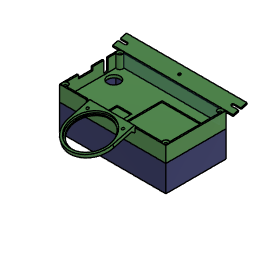
arcade console v12 (Autodesk Fusion 360 archive; units mm, degrees)
design "scatolo"
Autodesk Fusion 360 part; units mm, degrees
(part 1 of 3)
sketch "Schizzo1" plane through (0, 0, 0) normal (0, 0, 1) x (1, 0, 0)
  line L0 (-75, 42.5) -> (75, 42.5)
  line L1 (75, 42.5) -> (75, -42.5)
  line L2 (75, -42.5) -> (-75, -42.5)
  line L3 (-75, -42.5) -> (-75, 42.5)
  line L4 (0, 42.5) -> (0, -42.5) construction
  dimension "d1" = 150
  dimension "d2" = 85
  constraint horizontal L0
  constraint vertical L1
  constraint horizontal L2
  constraint vertical L3
  constraint midpoint L0 L4.start
  constraint midpoint L2 L4.end
  constraint midpoint origin L4
  measures "d1" distance of L0.start L0.end
  measures "d2" distance of L0.start L2.end
extrude "Estrusione1" add sketch "Schizzo1" along normal blind 2 makes body 1
sketch "Schizzo2" plane through (0, 0, 2) normal (0, 0, 1) x (-1, 0, 0)
  line L0 (75, 42.5) -> (-75, 42.5)
  line L1 (-75, 42.5) -> (-75, -42.5)
  line L2 (-75, -42.5) -> (75, -42.5)
  line L3 (75, -42.5) -> (75, 42.5)
  line L4 (75, -42.5) -> (-75, -42.5)
  line L5 (-75, -42.5) -> (-75, 42.5)
  line L6 (-75, 42.5) -> (75, 42.5)
  line L7 (75, 42.5) -> (75, -42.5)
  circle A0 centre (71, -38.5) radius 1
  circle A1 centre (71, -38.5) radius 4
  circle A2 centre (-71, -38.5) radius 1
  circle A3 centre (-71, -38.5) radius 4
  circle A4 centre (71, 38.5) radius 1
  circle A5 centre (71, 38.5) radius 4
  circle A6 centre (-71, 38.5) radius 1
  circle A7 centre (-71, 38.5) radius 4
  line L8 (-73, -40.5) -> (-73, 40.5)
  line L9 (-73, 40.5) -> (73, 40.5)
  line L10 (73, 40.5) -> (73, -40.5)
  line L11 (73, -40.5) -> (-73, -40.5)
  point P0 (-67, -42.5)
  point P1 (-67, -42.5)
  point P2 (75, 34.5)
  point P3 (75, 34.5)
  point P4 (-67, 34.5)
  point P5 (-67, 34.5)
  dimension "d5" = 2
  dimension "d6" = 4
  dimension "d7" = 4
  dimension "d8" = 8
  dimension "d11" = -142
  dimension "d12" = 77
  dimension "d13" = 2
  constraint horizontal L4
  constraint vertical L5
  constraint horizontal L6
  constraint vertical L7
  constraint coincident L0.end L1.start
  constraint coincident L2.end L3.start
  constraint concentric A0 A1
  measures "d5" diameter of A0
  measures "d6" distance of L7 A0.centre
  measures "d7" distance of L4 A0.centre
  measures "d8" diameter of A1
extrude "Estrusione2" add sketch "Schizzo2" along normal blind 35 contours L0 L3 L6 L7 A5 | L0 L6 A5 A7 L9 | A5 L9 L10 | L3 L7 A1 A5 L10 | L0 L1 L5 L6 A7 | A7 L8 L9 | A5 L9 L10 | A1 L10 L11 | L2 L3 L4 L7 A1 | A7 L8 L9 | L1 L5 A3 A7 L8 | A1 L10 L11 | L2 L4 A1 A3 L11 | L1 L2 L4 L5 A3 | A3 L8 L11 | A3 L8 L11 bodies 1
sketch "Schizzo3" plane through (0, 0, 2) normal (0, 0, 1) x (-1, 0, 0)
  arc A0 (-73, 35.0359) -> (-67.5359, 40.5) centre (-71, 38.5) ccw
  line L0 (63.75, -38.5) -> (-63.75, -38.5)
  line L1 (-63.75, -38.5) -> (-63.75, 38.5)
  line L2 (-63.75, 38.5) -> (63.75, 38.5)
  line L3 (63.75, 38.5) -> (63.75, -38.5)
  arc A1 (-67.5359, -40.5) -> (-73, -35.0359) centre (-71, -38.5) ccw
  line L4 (-73, 35.0359) -> (-73, -35.0359)
  arc A2 (67.5359, 40.5) -> (73, 35.0359) centre (71, 38.5) ccw
  line L5 (67.5359, 40.5) -> (-67.5359, 40.5)
  line L6 (-67.5359, -40.5) -> (67.5359, -40.5)
  arc A3 (73, -35.0359) -> (67.5359, -40.5) centre (71, -38.5) ccw
  line L7 (73, -35.0359) -> (73, 35.0359)
  line L8 (0, -38.5) -> (0, 38.5) construction
  dimension "d16" = 127.5
  dimension "d17" = 77
  constraint horizontal L0
  constraint vertical L1
  constraint horizontal L2
  constraint vertical L3
  constraint midpoint L0 L8.start
  constraint midpoint L2 L8.end
  constraint midpoint origin L8
  measures "d16" distance of L0.start L0.end
  measures "d17" distance of L0.start L2.end
extrude "Estrusione3" add sketch "Schizzo3" along normal blind 2 bodies 1
sketch "Schizzo4" plane through (0, 40.5, 0) normal (0, -1, 0) x (1, 0, 0)
  line L0 (-67.5359, 4) -> (67.5359, 4)
  line L1 (67.5359, 4) -> (67.5359, 37)
  line L2 (67.5359, 37) -> (-67.5359, 37)
  line L3 (-67.5359, 37) -> (-67.5359, 4)
  circle A0 centre (48.6233, 33.35) radius 3.65
  line L4 (44.9733, 33.35) -> (52.2733, 33.35)
  line L5 (52.2733, 33.35) -> (52.2733, 37)
  line L6 (52.2733, 37) -> (44.9733, 37)
  line L7 (44.9733, 37) -> (44.9733, 33.35)
  dimension "d20" = 7.3
  constraint horizontal L4
  constraint vertical L5
  constraint horizontal L6
  constraint vertical L7
  constraint tangent A0 L7
  constraint tangent A0 L6
  constraint tangent A0 L5
  constraint midpoint A0.centre L4
  constraint collinear L2 L6
  measures "d20" diameter of A0
extrude "Estrusione4" cut sketch "Schizzo4" against normal blind 16.479 contours L2 A0 L6 L7 | L2 A0 L5 L6 | A0 L4 | A0 L4 bodies 1
sketch "Schizzo5" plane through (0, 0, 37) normal (0, 0, 1) x (-1, 0, 0)
  line L0 (-52.2733, -42.5) -> (-52.2733, -40.5)
  line L1 (-52.2733, -40.5) -> (-67.5359, -40.5)
  arc A0 (-67.5359, -40.5) -> (-73, -35.0359) centre (-71, -38.5) ccw
  line L2 (-73, -35.0359) -> (-73, 35.0359)
  arc A1 (-73, 35.0359) -> (-67.5359, 40.5) centre (-71, 38.5) ccw
  line L3 (-67.5359, 40.5) -> (67.5359, 40.5)
  arc A2 (67.5359, 40.5) -> (73, 35.0359) centre (71, 38.5) ccw
  line L4 (73, 35.0359) -> (73, -35.0359)
  arc A3 (73, -35.0359) -> (67.5359, -40.5) centre (71, -38.5) ccw
  line L5 (67.5359, -40.5) -> (-44.9733, -40.5)
  line L6 (-44.9733, -40.5) -> (-44.9733, -42.5)
  line L7 (-44.9733, -42.5) -> (75, -42.5)
  line L8 (75, -42.5) -> (75, 42.5)
  line L9 (75, 42.5) -> (-75, 42.5)
  line L10 (-75, 42.5) -> (-75, -42.5)
  line L11 (-75, -42.5) -> (-52.2733, -42.5)
  circle A4 centre (-71, 38.5) radius 1
  circle A5 centre (71, -38.5) radius 1
  circle A6 centre (71, 38.5) radius 1
  circle A7 centre (-71, -38.5) radius 1
  circle A8 centre (-71, 38.5) radius 2
  circle A9 centre (71, 38.5) radius 2
  circle A10 centre (71, -38.5) radius 2
  circle A11 centre (-71, -38.5) radius 2
  line L12 (-44.9733, -42.5) -> (-52.2733, -42.5)
  dimension "d23" = 4
  dimension "d24" = 4
  dimension "d25" = 4
  dimension "d26" = 4
  constraint concentric A1 A8
  constraint concentric A2 A9
  constraint concentric A3 A10
  constraint concentric A0 A11
  constraint coincident L6.end L7.start
  constraint coincident L0.start L11.end
  measures "d23" diameter of A8
  measures "d24" diameter of A9
  measures "d25" diameter of A10
  measures "d26" diameter of A11
extrude "Estrusione1'" add sketch "Schizzo5" along normal blind 2 separate body contours L0 L1 A0 L2 A1 L3 A2 L4 A3 L5 L6 L7 L8 L9 L10 L11 | L0 L1 A0 L2 A1 L3 A2 L4 A3 L5 L6 L12 makes body 2 in component "sopra"
sketch "Schizzo6" plane through (0, 0, 39) normal (0, 0, 1) x (-1, 0, 0)
  circle A0 centre (-71, 38.5) radius 2
  circle A1 centre (-71, -38.5) radius 2
  circle A2 centre (71, -38.5) radius 2
  circle A3 centre (71, 38.5) radius 2
  line L0 (75, -42.5) -> (75, 42.5)
  line L1 (75, 42.5) -> (-75, 42.5)
  line L2 (-75, 42.5) -> (-75, -42.5)
  line L3 (-75, -42.5) -> (75, -42.5)
  line L4 (-52.2733, -42.5) -> (-52.2733, -40.5)
  line L5 (-52.2733, -40.5) -> (-67.5359, -40.5)
  arc A4 (-67.5359, -40.5) -> (-73, -35.0359) centre (-71, -38.5) ccw
  line L6 (-73, -35.0359) -> (-73, 35.0359)
  arc A5 (-73, 35.0359) -> (-67.5359, 40.5) centre (-71, 38.5) ccw
  line L7 (-67.5359, 40.5) -> (67.5359, 40.5)
  arc A6 (67.5359, 40.5) -> (73, 35.0359) centre (71, 38.5) ccw
  line L8 (73, 35.0359) -> (73, -35.0359)
  arc A7 (73, -35.0359) -> (67.5359, -40.5) centre (71, -38.5) ccw
  line L9 (67.5359, -40.5) -> (-44.9733, -40.5)
  line L10 (-44.9733, -40.5) -> (-44.9733, -42.5)
  line L11 (-44.9733, -42.5) -> (75, -42.5)
  line L12 (75, -42.5) -> (75, 42.5)
  line L13 (75, 42.5) -> (-75, 42.5)
  line L14 (-75, 42.5) -> (-75, -42.5)
  line L15 (-75, -42.5) -> (-52.2733, -42.5)
  circle A8 centre (-71, 38.5) radius 1
  circle A9 centre (71, -38.5) radius 1
  circle A10 centre (71, 38.5) radius 1
  circle A11 centre (-71, -38.5) radius 1
  line L16 (-52.2733, -40.5) -> (-44.9733, -40.5)
  line L17 (-44.9733, -40.5) -> (-44.9733, -42.5)
  line L18 (-44.9733, -42.5) -> (-52.2733, -42.5)
  line L19 (-52.2733, -42.5) -> (-52.2733, -40.5)
  constraint horizontal L16
  constraint vertical L17
  constraint horizontal L18
  constraint vertical L19
  constraint coincident L10.end L11.start
  constraint coincident L4.end L5.start
extrude "Estrusione2'" add sketch "Schizzo6" along normal blind 20 contours L0 L1 L2 L3 L4 L5 A4 L6 A5 L7 A6 L8 A7 L9 L10 L11 L12 L13 L14 L15 L17 L19 | L3 L4 L10 L16 L17 L18 L19 bodies 2 in component "sopra"
sketch "Schizzo7" plane through (0, 0, 39) normal (0, 0, 1) x (-1, 0, 0)
  arc A0 (73, -35.0359) -> (67.5359, -40.5) centre (71, -38.5) ccw
  line L0 (73, -35.0359) -> (73, 35.0359)
  arc A1 (67.5359, 40.5) -> (73, 35.0359) centre (71, 38.5) ccw
  line L1 (67.5359, 40.5) -> (-67.5359, 40.5)
  arc A2 (-73, 35.0359) -> (-67.5359, 40.5) centre (-71, 38.5) ccw
  line L2 (-73, 35.0359) -> (-73, -35.0359)
  arc A3 (-67.5359, -40.5) -> (-73, -35.0359) centre (-71, -38.5) ccw
  line L3 (-67.5359, -40.5) -> (67.5359, -40.5)
  circle A4 centre (60, -19) radius 9
  dimension "d31" = 18
  measures "d31" diameter of A4
extrude "Estrusione3'" cut sketch "Schizzo7" against normal blind 8.932 contours A4 bodies 2 in component "sopra"
sketch "Schizzo8" plane through (0, 40.5, 0) normal (0, -1, 0) x (1, 0, 0)
  line L0 (-67.5359, 39) -> (67.5359, 39)
  line L1 (67.5359, 39) -> (67.5359, 59)
  line L2 (67.5359, 59) -> (-67.5359, 59)
  line L3 (-67.5359, 59) -> (-67.5359, 39)
sketch "Schizzo9" plane through (0, 0, 39) normal (0, 0, 1) x (-1, 0, 0)
  circle A0 centre (60, -19) radius 9
  arc A1 (73, -35.0359) -> (67.5359, -40.5) centre (71, -38.5) ccw
  line L0 (73, -35.0359) -> (73, 35.0359)
  arc A2 (67.5359, 40.5) -> (73, 35.0359) centre (71, 38.5) ccw
  line L1 (67.5359, 40.5) -> (-67.5359, 40.5)
  arc A3 (-73, 35.0359) -> (-67.5359, 40.5) centre (-71, 38.5) ccw
  line L2 (-73, 35.0359) -> (-73, -35.0359)
  arc A4 (-67.5359, -40.5) -> (-73, -35.0359) centre (-71, -38.5) ccw
  line L3 (-67.5359, -40.5) -> (67.5359, -40.5)
  circle A5 centre (-23.6081, -24.9772) radius 0.254
  line L4 (-46.4381, -12.0232) -> (-46.4381, 20.7428)
  line L5 (22.1119, 25.8228) -> (22.1119, -27.5557)
  circle A6 centre (0.7459, -24.9772) radius 0.254
  circle A7 centre (-15.9881, 23.2828) radius 0.254
  circle A8 centre (-26.1481, -24.9772) radius 0.254
  circle A9 centre (-33.7681, 23.2828) radius 0.254
  circle A10 centre (-41.3881, -24.9772) radius 0.254
  circle A11 centre (-13.4481, 23.2828) radius 0.254
  circle A12 centre (-28.6881, 23.2828) radius 0.254
  circle A13 centre (-5.8281, 23.2828) radius 0.254
  circle A14 centre (-31.2281, 23.2828) radius 0.254
  line L6 (-43.9581, 25.8228) -> (22.1119, 25.8228)
  line L7 (-43.9581, 25.8228) -> (-43.9581, 23.2828)
  circle A15 centre (-1.7941, -24.9772) radius 0.254
  line L8 (-43.9581, -14.5632) -> (-46.4381, -12.0232)
  circle A16 centre (-38.8481, 23.2828) radius 0.254
  circle A17 centre (-11.9541, -24.9772) radius 0.254
  circle A18 centre (-10.9081, 23.2828) radius 0.254
  circle A19 centre (-9.4141, -24.9772) radius 0.254
  circle A20 centre (3.2859, -24.9772) radius 0.254
  circle A21 centre (-18.5281, 23.2828) radius 0.254
  circle A22 centre (-19.5741, -24.9772) radius 0.254
  line L9 (-46.4381, 20.7428) -> (-43.9581, 23.2828)
  circle A23 centre (-23.6081, 23.2828) radius 0.254
  circle A24 centre (-14.4941, -24.9772) radius 0.254
  circle A25 centre (-4.3341, -24.9772) radius 0.254
  line L10 (-43.9581, -25.9909) -> (-42.3933, -27.5557)
  line L11 (-42.3933, -27.5557) -> (22.1119, -27.5557)
  circle A26 centre (-31.2281, -24.9772) radius 0.254
  circle A27 centre (-6.8741, -24.9772) radius 0.254
  circle A28 centre (-36.3081, -24.9772) radius 0.254
  circle A29 centre (-17.0341, -24.9772) radius 0.254
  circle A30 centre (-41.3881, 23.2828) radius 0.254
  circle A31 centre (-38.8481, -24.9772) radius 0.254
  circle A32 centre (-28.6881, -24.9772) radius 0.254
  circle A33 centre (-33.7681, -24.9772) radius 0.254
  circle A34 centre (-36.3081, 23.2828) radius 0.254
  circle A35 centre (8.1419, 23.2828) radius 1.5875
  circle A36 centre (-43.9581, -9.7372) radius 1.5875
  circle A37 centre (-21.0681, 23.2828) radius 0.254
  circle A38 centre (6.8419, -24.9772) radius 1.5875
  circle A39 centre (-43.9581, 18.2028) radius 1.5875
  circle A40 centre (-8.3681, 23.2828) radius 0.254
  line L12 (-43.9581, -25.9909) -> (-43.9581, -14.5632)
  circle A41 centre (-45.7728, -24.3932) radius 0.254
  line L13 (-68.6028, -11.4392) -> (-68.6028, 21.3268)
  line L14 (-0.0528, 26.4068) -> (-0.0528, -26.9717)
  circle A42 centre (-21.4188, -24.3932) radius 0.254
  circle A43 centre (-38.1528, 23.8668) radius 0.254
  circle A44 centre (-48.3128, -24.3932) radius 0.254
  circle A45 centre (-55.9328, 23.8668) radius 0.254
  circle A46 centre (-63.5528, -24.3932) radius 0.254
  circle A47 centre (-35.6128, 23.8668) radius 0.254
  circle A48 centre (-50.8528, 23.8668) radius 0.254
  circle A49 centre (-27.9928, 23.8668) radius 0.254
  circle A50 centre (-53.3928, 23.8668) radius 0.254
  line L15 (-66.1228, 26.4068) -> (-0.0528, 26.4068)
  line L16 (-66.1228, 26.4068) -> (-66.1228, 23.8668)
  circle A51 centre (-23.9588, -24.3932) radius 0.254
  line L17 (-66.1228, -13.9792) -> (-68.6028, -11.4392)
  circle A52 centre (-61.0128, 23.8668) radius 0.254
  circle A53 centre (-34.1188, -24.3932) radius 0.254
  circle A54 centre (-33.0728, 23.8668) radius 0.254
  circle A55 centre (-31.5788, -24.3932) radius 0.254
  circle A56 centre (-18.8788, -24.3932) radius 0.254
  circle A57 centre (-40.6928, 23.8668) radius 0.254
  circle A58 centre (-41.7388, -24.3932) radius 0.254
  line L18 (-68.6028, 21.3268) -> (-66.1228, 23.8668)
  circle A59 centre (-45.7728, 23.8668) radius 0.254
  circle A60 centre (-36.6588, -24.3932) radius 0.254
  circle A61 centre (-26.4988, -24.3932) radius 0.254
  line L19 (-66.1228, -25.4069) -> (-64.558, -26.9717)
  line L20 (-64.558, -26.9717) -> (-0.0528, -26.9717)
  circle A62 centre (-53.3928, -24.3932) radius 0.254
  circle A63 centre (-29.0388, -24.3932) radius 0.254
  circle A64 centre (-58.4728, -24.3932) radius 0.254
  circle A65 centre (-39.1988, -24.3932) radius 0.254
  circle A66 centre (-63.5528, 23.8668) radius 0.254
  circle A67 centre (-61.0128, -24.3932) radius 0.254
  circle A68 centre (-50.8528, -24.3932) radius 0.254
  circle A69 centre (-55.9328, -24.3932) radius 0.254
  circle A70 centre (-58.4728, 23.8668) radius 0.254
  circle A71 centre (-14.0228, 23.8668) radius 1.5875
  circle A72 centre (-66.1228, -9.1532) radius 1.5875
  circle A73 centre (-43.2328, 23.8668) radius 0.254
  circle A74 centre (-15.3228, -24.3932) radius 1.5875
  circle A75 centre (-66.1228, 18.7868) radius 1.5875
  circle A76 centre (-30.5328, 23.8668) radius 0.254
  line L21 (-66.1228, -25.4069) -> (-66.1228, -13.9792)
  dimension "d34" = 50.8881
  measures "d34" distance of L0 L5
extrude "Estrusione4'" add sketch "Schizzo9" along normal blind 2 contours A1 L0 A2 L1 A3 L2 A4 L3 | L5 L6 L10 L11 L14 L20 | A6 | A20 | A35 | A38 bodies 2 in component "sopra"
sketch "Schizzo10" plane through (0, 0, 39) normal (0, 0, 1) x (-1, 0, 0)
  line L0 (-0.0528, -26.9717) -> (-0.0528, 26.4068)
  line L1 (-0.0528, 26.4068) -> (-66.1228, 26.4068)
  line L2 (-66.1228, 26.4068) -> (-66.1228, 23.8668)
  line L3 (-66.1228, 23.8668) -> (-68.6028, 21.3268)
  line L4 (-68.6028, 21.3268) -> (-68.6028, -11.4392)
  line L5 (-68.6028, -11.4392) -> (-66.1228, -13.9792)
  line L6 (-66.1228, -13.9792) -> (-66.1228, -25.4069)
  line L7 (-66.1228, -25.4069) -> (-64.558, -26.9717)
  line L8 (-64.558, -26.9717) -> (-0.0528, -26.9717)
  line L9 (0.4472, 26.9068) -> (-66.6228, 26.9068)
  line L10 (-66.6228, 26.9068) -> (-66.6228, 24.0704)
  line L11 (-66.6228, 24.0704) -> (-69.1028, 21.5304)
  line L12 (-69.1028, 21.5304) -> (-69.1028, -11.6428)
  line L13 (-69.1028, -11.6428) -> (-66.6228, -14.1828)
  line L14 (-66.6228, -14.1828) -> (-66.6228, -25.614)
  line L15 (-66.6228, -25.614) -> (-64.7651, -27.4717)
  line L16 (-64.7651, -27.4717) -> (0.4472, -27.4717)
  line L17 (0.4472, -27.4717) -> (0.4472, 26.9068)
  dimension "d37" = 0.5
extrude "Estrusione5" cut sketch "Schizzo10" along normal blind 34.396 bodies 2 in component "sopra"
ref_plane "Piano di lavoro1" through (0, 0, 48) normal (-1, 0, 0) x (0, -1, 0)
sketch "Schizzo12" plane through (0, 0, 0) normal (-1, 0, 0) x (0, -1, 0)
  line L0 (-42.5, 37) -> (42.5, 37) construction
  line L1 (42.5, 37) -> (42.5, 59) construction
  line L2 (42.5, 59) -> (-42.5, 59) construction
  line L3 (-42.5, 59) -> (-42.5, 37) construction
  line L4 (-42.5, 59) -> (-61.8185, 64.1764)
  line L5 (-42.5, 59) -> (-22.5, 59) construction
  line L6 (-61.8185, 64.1764) -> (-62.3362, 62.2445)
  line L7 (-62.3362, 62.2445) -> (-42.5, 56.9294)
  line L8 (-42.5, 59) -> (-42.5, 56.9294)
  dimension "d40" = 165
  dimension "d41" = 20
  dimension "d42" = 2
  constraint horizontal L5
  constraint coincident L2.end L3.start
  constraint perpendicular L4 L6
  constraint perpendicular L6 L7
  constraint perpendicular L2 L8
  constraint coincident L3 L7.end
  measures "d40" angle of L4 L5
  measures "d41" distance of L2.end L4.end
  measures "d42" distance of L4.end L6.end
extrude "Estrusione6" add sketch "Schizzo12" along normal mid plane 170 bodies 2 in component "sopra"
sketch "Schizzo13" plane through (0, -11.903, 44.4227) normal (0, -0.258819, 0.965926) x (1, 0, 0)
  line L0 (85, 76.3222) -> (-85, 76.3222)
  line L1 (-85, 76.3222) -> (-85, 56.3222)
  line L2 (-85, 56.3222) -> (-75, 56.3222)
  line L3 (-75, 56.3222) -> (75, 56.3222)
  line L4 (75, 56.3222) -> (85, 56.3222)
  line L5 (85, 56.3222) -> (85, 76.3222)
  line L6 (-85, 76.3222) -> (85, 76.3222) construction
  line L7 (-85, 65.8222) -> (85, 65.8222) construction
  circle A0 centre (-75, 65.8222) radius 1.75
  line L8 (-85, 67.5722) -> (-75, 67.5722)
  line L9 (-75, 67.5722) -> (-75, 64.0722)
  line L10 (-75, 64.0722) -> (-85, 64.0722)
  line L11 (-85, 64.0722) -> (-85, 67.5722)
  circle A1 centre (0, 65.8222) radius 1.75
  circle A2 centre (75, 65.8222) radius 1.75
  line L12 (85, 67.5722) -> (75, 67.5722)
  line L13 (75, 67.5722) -> (75, 64.0722)
  line L14 (75, 64.0722) -> (85, 64.0722)
  line L15 (85, 64.0722) -> (85, 67.5722)
  dimension "d45" = 9.5
  dimension "d46" = 3.5
  dimension "d47" = 3.5
  dimension "d48" = 3.5
  dimension "d49" = 10
  dimension "d50" = 10
  constraint coincident L1 L7.start
  constraint coincident L5 L7.end
  constraint perpendicular L5 L7
  constraint coincident L7 A0.centre
  constraint horizontal L8
  constraint vertical L9
  constraint horizontal L10
  constraint vertical L11
  constraint midpoint L7 A1.centre
  constraint coincident L7 A2.centre
  constraint horizontal L12
  constraint vertical L13
  constraint horizontal L14
  constraint vertical L15
  constraint collinear L5 L15
  constraint collinear L1 L11
  constraint midpoint A2.centre L13
  constraint midpoint A0.centre L9
  constraint tangent A0 L8
  constraint tangent A2 L12
  measures "d45" distance of L2 L7
  measures "d46" diameter of A0
  measures "d47" diameter of A1
  measures "d48" diameter of A2
  measures "d49" distance of L8.start L8.end
  measures "d50" distance of L12.start L12.end
extrude "Estrusione7" cut sketch "Schizzo13" against normal blind 2.904 contours L5 A2 L12 L14 L15 | L1 A0 L8 L10 L11 | A2 L13 | A2 L13 | A0 L9 | A0 L9 | A1 bodies 2 in component "sopra"
sketch "Schizzo14" plane through (0, 0, 0) normal (-1, 0, 0) x (0, -1, 0)
  line L0 (43.4059, 62.3807) -> (42.5, 59)
  line L1 (43.4059, 62.3807) -> (46.9059, 62.3807) construction
  line L2 (42.5, 37) -> (-42.5, 37) construction
  line L3 (-42.5, 37) -> (-42.5, 56.9294) construction
  line L4 (-42.5, 56.9294) -> (-42.5, 59) construction
  line L5 (-42.5, 59) -> (42.5, 59) construction
  line L6 (42.5, 59) -> (42.5, 37) construction
  line L7 (43.4059, 62.3807) -> (104.2592, 46.0751)
  line L8 (43.4059, 62.3807) -> (106.4059, 62.3807) construction
  line L9 (104.2592, 46.0751) -> (102.9651, 41.2455)
  line L10 (102.9651, 41.2455) -> (42.5, 57.4471)
  line L11 (42.5, 59) -> (42.5, 57.4471)
  line L12 (-34.5, 59) -> (-40.5, 59) construction
  line L13 (-35.0359, 59) -> (35.0359, 59) construction
  line L14 (40.5, 59) -> (34.5, 59) construction
  line L15 (40.5, 59) -> (34.5, 59) construction
  line L16 (35.0359, 59) -> (-35.0359, 59) construction
  line L17 (-34.5, 59) -> (-40.5, 59) construction
  line L18 (36.5, 59) -> (40.5, 59) construction
  line L19 (-40.5, 59) -> (-36.5, 59) construction
  line L20 (-40.5, 59) -> (-36.5, 59) construction
  line L21 (36.5, 59) -> (40.5, 59) construction
  line L22 (-42.5, 59) -> (42.5, 59) construction
  line L23 (42.5, 59) -> (-42.5, 59) construction
  line L24 (40.5, 59) -> (43.4059, 62.3807)
  line L25 (42.5, 59) -> (40.5, 59)
  dimension "d53" = 105
  dimension "d54" = 3.5
  dimension "d55" = 15
  dimension "d56" = 63
  dimension "d57" = 5
  constraint horizontal L1
  constraint coincident L0.end L5.end
  constraint horizontal L8
  constraint perpendicular L7 L9
  constraint perpendicular L9 L10
  constraint perpendicular L5 L11
  constraint coincident L6 L10.end
  constraint coincident L14.start L15.start
  measures "d53" angle of L0 L1
  measures "d54" distance of L0.start L0.end
  measures "d55" angle of L7 L8
  measures "d56" distance of L0.start L7.end
  measures "d57" distance of L7.end L9.end
extrude "Estrusione8" add sketch "Schizzo14" along normal mid plane 63 bodies 2 in component "sopra"
chamfer "Smusso1" distance 5 angle 45 1 edges at (0, -42.5, 57.4471) on bodies 2 in component "sopra"
sketch "Schizzo15" plane through (0, -18.5028, 69.0535) normal (0, -0.258819, 0.965926) x (1, 0, 0)
  line L0 (31.5, -25.7815) -> (-31.5, -25.7815)
  line L1 (-31.5, -25.7815) -> (-31.5, -88.7815)
  line L2 (-31.5, -88.7815) -> (31.5, -88.7815)
  line L3 (31.5, -88.7815) -> (31.5, -25.7815)
  circle A0 centre (0, -57.2815) radius 28.5
  line L4 (-31.5, -85.7815) -> (31.5, -85.7815) construction
  line L5 (31.5, -85.7815) -> (31.5, -88.7815) construction
  line L6 (31.5, -88.7815) -> (-31.5, -88.7815) construction
  line L7 (-31.5, -88.7815) -> (-31.5, -85.7815) construction
  line L8 (-63.75, -36.6705, -59.593) -> (63.75, -36.6705, -59.593) construction
  line L9 (0, -85.7815) -> (0, -112) construction
  dimension "d61" = 57
  dimension "d62" = 3
  constraint horizontal L4
  constraint vertical L5
  constraint horizontal L6
  constraint vertical L7
  constraint collinear L2 L6
  constraint tangent A0 L4
  constraint collinear L3 L5
  constraint collinear L1 L7
  constraint midpoint L4 L9.start
  constraint perpendicular L4 L9
  constraint coincident A0.centre L9
  measures "d61" diameter of A0
  measures "d62" distance of L4.start L1.end
extrude "Estrusione9" cut sketch "Schizzo15" against normal blind 3 contours A0 bodies 2 in component "sopra"
sketch "Schizzo16" plane through (0, -17.7264, 66.1557) normal (0, -0.258819, 0.965926) x (1, 0, 0)
  circle A0 centre (0, -57.2815) radius 28.5
  circle A1 centre (0, -57.2815) radius 26.5
  dimension "d65" = 53
  constraint concentric A0 A1
  measures "d65" diameter of A1
extrude "Estrusione10" cut sketch "Schizzo16" against normal blind 2.232 contours A1 bodies 2 in component "sopra"
sketch "Schizzo17" plane through (0, 0, 41) normal (0, 0, 1) x (-1, 0, 0)
  line L0 (0.4472, -27.4717) -> (-64.7651, -27.4717)
  line L1 (-64.7651, -27.4717) -> (-66.6228, -25.614)
  line L2 (-66.6228, -25.614) -> (-66.6228, -14.1828)
  line L3 (-66.6228, -14.1828) -> (-69.1028, -11.6428)
  line L4 (-69.1028, -11.6428) -> (-69.1028, 21.5304)
  line L5 (-69.1028, 21.5304) -> (-66.6228, 24.0704)
  line L6 (-66.6228, 24.0704) -> (-66.6228, 26.9068)
  line L7 (-66.6228, 26.9068) -> (0.4472, 26.9068)
  line L8 (0.4472, 26.9068) -> (0.4472, -27.4717)
  circle A0 centre (60, -19) radius 9
  line L9 (-73, 35.0359) -> (-73, -35.0359)
  arc A1 (-67.5359, -40.5) -> (-73, -35.0359) centre (-71, -38.5) ccw
  line L10 (-67.5359, -40.5) -> (67.5359, -40.5)
  arc A2 (73, -35.0359) -> (67.5359, -40.5) centre (71, -38.5) ccw
  line L11 (73, -35.0359) -> (73, 35.0359)
  arc A3 (67.5359, 40.5) -> (73, 35.0359) centre (71, 38.5) ccw
  line L12 (67.5359, 40.5) -> (-67.5359, 40.5)
  arc A4 (-73, 35.0359) -> (-67.5359, 40.5) centre (-71, 38.5) ccw
  line L13 (26.4472, 9.9068) -> (5.4472, 9.9068)
  line L14 (5.4472, 9.9068) -> (5.4472, 26.9068)
  line L15 (5.4472, 26.9068) -> (26.4472, 26.9068)
  line L16 (26.4472, 26.9068) -> (26.4472, 9.9068)
  dimension "d68" = 5
  dimension "d69" = 21
  dimension "d70" = 17
  constraint horizontal L13
  constraint vertical L14
  constraint horizontal L15
  constraint vertical L16
  constraint collinear L7 L15
  measures "d68" distance of L8 L14
  measures "d69" distance of L13.start L13.end
  measures "d70" distance of L13.start L15.end
extrude "Estrusione11" cut sketch "Schizzo17" against normal blind 2 contours L13 L14 L15 L16 bodies 2 in component "sopra"
sketch "Schizzo18" plane through (0, -42.5, 0) normal (0, -1, 0) x (1, 0, 0)
  line L0 (-31.5, 52.4471) -> (-31.5, 59)
  line L1 (-31.5, 59) -> (-75, 59)
  line L2 (-75, 59) -> (-75, 37)
  line L3 (-75, 37) -> (75, 37)
  line L4 (75, 37) -> (75, 59)
  line L5 (75, 59) -> (31.5, 59)
  line L6 (31.5, 59) -> (31.5, 52.4471)
  line L7 (31.5, 52.4471) -> (-31.5, 52.4471)
  circle A0 centre (-35.6271, 49) radius 1.5
  line L8 (-37.1271, 59) -> (-34.1271, 59)
  line L9 (-34.1271, 59) -> (-34.1271, 49)
  line L10 (-34.1271, 49) -> (-37.1271, 49)
  line L11 (-37.1271, 49) -> (-37.1271, 59)
  dimension "d73" = 3
  dimension "d74" = 3
  dimension "d75" = 10
  constraint horizontal L8
  constraint vertical L9
  constraint horizontal L10
  constraint vertical L11
  constraint collinear L1 L8
  constraint midpoint A0.centre L10
  measures "d73" diameter of A0
  measures "d74" distance of L8.start L8.end
  measures "d75" distance of L8.start L10.end
extrude "Estrusione12" cut sketch "Schizzo18" against normal blind 5.663 contours L1 A0 L8 L9 L11 | A0 L10 | A0 L10 bodies 2 in component "sopra"
fillet "Raccordo1" radius 31.5 2 edges at (-31.5, -103.6121, 43.6603) (31.5, -103.6121, 43.6603) on bodies 2 in component "sopra"
sketch "Schizzo19" plane through (0, -18.5028, 69.0535) normal (0, -0.258819, 0.965926) x (1, 0, 0)
  arc A0 (-31.5, -57.2815) -> (31.5, -57.2815) centre (0, -57.2815) ccw
  line L0 (31.5, -57.2815) -> (31.5, -25.7815)
  line L1 (31.5, -25.7815) -> (-31.5, -25.7815)
  line L2 (-31.5, -25.7815) -> (-31.5, -57.2815)
  circle A1 centre (0, -57.2815) radius 28.5
  circle A2 centre (-25, -35.7815) radius 1.75
  circle A3 centre (25, -35.7815) radius 1.75
  line L3 (-25, -35.7815) -> (25, -35.7815)
  line L4 (0, -25.7815) -> (0, -35.7815)
  dimension "d80" = 3.5
  dimension "d81" = 3.5
  dimension "d82" = 50
  dimension "d85" = 10
  constraint coincident A2.centre L3.start
  constraint parallel L1 L3
  constraint midpoint L1 L4.start
  constraint midpoint L3 L4.end
  constraint vertical L4
  constraint coincident A3.centre L3.end
  measures "d80" diameter of A2
  measures "d81" diameter of A3
  measures "d82" distance of A2.centre A3.centre
  measures "d85" distance of L4.start L4.end
extrude "Estrusione13" cut sketch "Schizzo19" against normal blind 6.961 contours A2 | A3 bodies 2 in component "sopra"
copy_body "Corpo->Comp1" bodies 1 removing the originals makes body 3 in component "sotto"
chamfer "Smusso2" distance 1.8 angle 45 4 edges at (-69.1353, 37.7768, 59) (-69.1353, -39.2232, 59) (72.8647, 37.7768, 59) (72.8647, -39.2232, 59) on bodies 2 in component "sopra"
sketch "Schizzo20" plane through (-75, 0, 0) normal (-1, 0, 0) x (0, -1, 0)
  line L0 (-42.5, 37) -> (42.5, 37)
  line L1 (42.5, 37) -> (42.5, 59)
  line L2 (42.5, 59) -> (-42.5, 59)
  line L3 (-42.5, 59) -> (-42.5, 56.9294)
  line L4 (-42.5, 56.9294) -> (-42.5, 37)
  circle A0 centre (-20.9777, 44) radius 3
  line L5 (-23.9777, 59) -> (-17.9777, 59)
  line L6 (-17.9777, 59) -> (-17.9777, 44)
  line L7 (-17.9777, 44) -> (-23.9777, 44)
  line L8 (-23.9777, 44) -> (-23.9777, 59)
  line L9 (-26.9777, 59) -> (-14.9777, 59)
  line L10 (-14.9777, 59) -> (-14.9777, 47)
  line L11 (-14.9777, 47) -> (-26.9777, 47)
  line L12 (-26.9777, 47) -> (-26.9777, 59)
  dimension "d87" = 6
  dimension "d88" = 6
  dimension "d89" = 15
  dimension "d95" = 12
  dimension "d96" = 12
  constraint horizontal L5
  constraint vertical L6
  constraint horizontal L7
  constraint vertical L8
  constraint midpoint A0.centre L7
  constraint collinear L2 L5
  constraint horizontal L9
  constraint vertical L10
  constraint horizontal L11
  constraint vertical L12
  constraint midpoint L5 L9
  measures "d87" diameter of A0
  measures "d88" distance of L5.start L5.end
  measures "d89" distance of L5.start L7.end
  measures "d95" distance of L9.start L9.end
  measures "d96" distance of L9.start L11.end
extrude "Estrusione14" cut sketch "Schizzo20" against normal blind 5.067 contours L2 L5 L6 L8 L9 L11 | A0 L6 L11 | A0 L8 L11 | A0 L7 | A0 L7 bodies 2 in component "sopra"
sketch "Schizzo21" plane through (0, 0, 59) normal (0, 0, 1) x (-1, 0, 0)
  line L0 (73, -17.9777) -> (75, -17.9777)
  line L1 (75, -17.9777) -> (75, 42.5)
  line L2 (75, 42.5) -> (37.1271, 42.5)
  line L3 (37.1271, 42.5) -> (37.1271, 40.5)
  line L4 (37.1271, 40.5) -> (67.5359, 40.5)
  arc A0 (67.5359, 40.5) -> (73, 35.0359) centre (71, 38.5) ccw
  line L5 (73, 35.0359) -> (73, -17.9777)
  circle A1 centre (71, 38.5) radius 3.8
  line L6 (83.0164, -2.2982) -> (65.8423, -2.2982)
  line L7 (65.8423, -2.2982) -> (65.8423, 17.7018)
  line L8 (65.8423, 17.7018) -> (83.0164, 17.7018)
  line L9 (83.0164, 17.7018) -> (83.0164, -2.2982)
  dimension "d92" = 20
  constraint horizontal L6
  constraint vertical L7
  constraint horizontal L8
  constraint vertical L9
  measures "d92" distance of L6.start L8.end
extrude "Estrusione15" cut sketch "Schizzo21" against normal blind 5 contours L1 L5 L6 L8 bodies 2 in component "sopra"
component "sopra" placed x (1, 0, 0) y (0, 1, 0) z (0, 0, 1) at (0, 0, 0)
component "sotto" placed x (1, 0, 0) y (0, 1, 0) z (0, 0, 1) at (0, 0, 0)
equation "d40 = 180 deg - 15 deg"
equation "d53 = 90 deg + 15 deg"
equation "d56 = 57 mm + 6 mm"
equation "d58 = 57 mm + 6 mm"
equation "d79 = ( ( 57 + 6 ) / 2 ) * 1 mm"

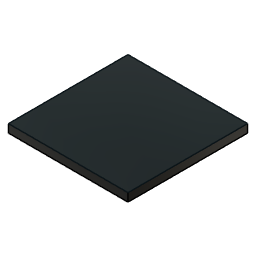
design "display 32x32"
Autodesk Fusion 360 part; units mm, degrees
sketch "Schizzo1" plane through (0, 0, 0) normal (0, 0, 1) x (1, 0, 0)
  line L0 (-96, 96) -> (96, 96)
  line L1 (96, 96) -> (96, -96)
  line L2 (96, -96) -> (-96, -96)
  line L3 (-96, -96) -> (-96, 96)
  line L4 (0, 96) -> (0, -96) construction
  dimension "d1" = 192
  dimension "d2" = 192
  constraint horizontal L0
  constraint vertical L1
  constraint horizontal L2
  constraint vertical L3
  constraint midpoint L0 L4.start
  constraint midpoint L2 L4.end
  constraint midpoint origin L4
  measures "d1" distance of L0.start L0.end
  measures "d2" distance of L0.start L2.end
extrude "Estrusione1" add sketch "Schizzo1" along normal blind 13.2 makes body 1
sketch "Schizzo2" plane through (0, 0, 13.2) normal (0, 0, 1) x (-1, 0, 0)
  line L0 (96, 96) -> (-96, 96)
  line L1 (-96, 96) -> (-96, -96)
  line L2 (-96, -96) -> (96, -96)
  line L3 (96, -96) -> (96, 96)
sketch "Schizzo3" plane through (0, 0, 0) normal (0, 0, -1) x (1, 0, 0)
  line L0 (96, 96) -> (-96, 96)
  line L1 (-96, 96) -> (-96, -96)
  line L2 (-96, -96) -> (96, -96)
  line L3 (96, -96) -> (96, 96)
  circle A0 centre (86.5, 0) radius 0.5
  circle A1 centre (-86.5, 0) radius 0.5
  line L4 (96, 0) -> (-96, 0) construction
  dimension "d5" = 1
  dimension "d6" = 1
  dimension "d7" = 9.5
  dimension "d8" = 9.5
  constraint midpoint L3 L4.start
  constraint midpoint L1 L4.end
  constraint coincident A0.centre L4
  constraint coincident A1.centre L4
  measures "d5" diameter of A0
  measures "d6" diameter of A1
  measures "d7" distance of L3 A0.centre
  measures "d8" distance of L1 A1.centre
hole "Foratura1" at (-86.5, 0, 0) at (86.5, 0, 0) direction (0, 0, 1) diameter 2.529 depth 6 tip angle 118 bodies 1
thread "Filettatura1" "ISO Metric profile 3.0 M3x0.5 6H" thread offset 0 thread depth 7.4
sketch "Schizzo4" plane through (0, 0, 13.2) normal (0, 0, 1) x (-1, 0, 0)
  circle A0 centre (-93, 93) radius 1.5
  line L0 (-96, 96) -> (-93, 96) construction
  line L1 (-93, 96) -> (-93, 93) construction
  line L2 (-93, 93) -> (-96, 93) construction
  line L3 (-96, 93) -> (-96, 96) construction
  point P0 (-96, 96)
  dimension "d14" = 3
  dimension "d15" = 3
  dimension "d16" = 3
  constraint horizontal L0
  constraint vertical L1
  constraint horizontal L2
  constraint vertical L3
  constraint coincident P0 L0.start
  constraint coincident A0.centre L1.end
  measures "d14" diameter of A0
  measures "d15" distance of P0 L0.end
  measures "d16" distance of P0 L2.end
extrude "Estrusione2" add sketch "Schizzo4" along normal blind 1 separate body makes body 2